Autodesk Fusion 360 part; units mm, degrees
note: some values were not read from the file. Chosen so that the rebuilt part matches the saved one: that a step has no effect.
(part 2 of 7)
  spline S227 degree 3 poles (-13.8567, 29.1803) (-14.5987, 29.1836) (-15.3407, 29.1895) (-16.0827, 29.1978) knots 0 0 0 0 1 1 1 1
  spline S228 degree 3 poles (-16.0827, 29.1978) (-16.65, 29.2012) (-16.65, 29.2012) (-17.2288, 29.2046) knots 0 0 0 0 1 1 1 1
  spline S229 degree 3 poles (-17.2288, 29.2046) (-18.1659, 29.2105) (-19.1029, 29.2194) (-20.04, 29.2289) knots 0 0 0 0 1 1 1 1
  spline S230 degree 3 poles (-20.04, 29.2289) (-20.2868, 29.9693) (-20.2868, 29.9693) (-20.5385, 30.7246) knots 0 0 0 0 1 1 1 1
  spline S231 degree 3 poles (-20.5385, 30.7246) (-20.374, 31.0537) (-20.2095, 31.3827) (-20.04, 31.7217) knots 0 0 0 0 1 1 1 1
  spline S232 degree 3 poles (-20.04, 31.7217) (-19.7109, 31.7217) (-19.3819, 31.7217) (-19.0429, 31.7217) knots 0 0 0 0 1 1 1 1
  spline S233 degree 3 poles (-19.0429, 31.7217) (-18.7888, 33.3829) (-18.5414, 35.045) (-18.295, 36.7073) knots 0 0 0 0 1 1 1 1
  spline S234 degree 3 poles (-18.295, 36.7073) (-18.2237, 37.1732) (-18.1524, 37.6392) (-18.0789, 38.1192) knots 0 0 0 0 1 1 1 1
  spline S235 degree 3 poles (-18.0789, 38.1192) (-17.6788, 40.8437) (-17.4748, 43.4272) (-17.5472, 46.1798) knots 0 0 0 0 1 1 1 1
  spline S236 degree 3 poles (-17.5472, 46.1798) (-17.5472, 46.8379) (-17.5472, 47.496) (-17.5472, 48.1741) knots 0 0 0 0 1 1 1 1
  spline S237 degree 3 poles (-17.5472, 48.1741) (-16.019, 48.9382) (-14.4225, 48.7239) (-12.7486, 48.7038) knots 0 0 0 0 1 1 1 1
  spline S238 degree 3 poles (18.3488, 14.7708) (18.5134, 14.2772) (18.6779, 13.7837) (18.8474, 13.2751) knots 0 0 0 0 1 1 1 1
  spline S239 degree 3 poles (18.8474, 13.2751) (19.1764, 13.5219) (19.5055, 13.7687) (19.8445, 14.023) knots 0 0 0 0 1 1 1 1
  spline S240 degree 3 poles (19.8445, 14.023) (21.7354, 14.9684) (23.2516, 15.2282) (25.3286, 14.7708) knots 0 0 0 0 1 1 1 1
  spline S241 degree 3 poles (25.3286, 14.7708) (26.9337, 13.5072) (27.674, 12.7203) (28.32, 10.7824) knots 0 0 0 0 1 1 1 1
  spline S242 degree 3 poles (28.32, 10.7824) (28.4814, 7.8759) (28.2625, 5.9661) (26.4192, 3.6779) knots 0 0 0 0 1 1 1 1
  spline S243 degree 3 poles (26.4192, 3.6779) (25.1645, 2.6742) (24.4352, 2.3869) (22.8358, 2.3069) knots 0 0 0 0 1 1 1 1
  spline S244 degree 3 poles (22.8358, 2.3069) (21.7141, 2.5562) (21.7141, 2.5562) (20.8416, 3.304) knots 0 0 0 0 1 1 1 1
  spline S245 degree 3 poles (20.8416, 3.304) (20.3431, 4.9867) (20.3431, 4.9867) (20.3431, 6.7939) knots 0 0 0 0 1 1 1 1
  spline S246 degree 3 poles (20.3431, 6.7939) (21.2467, 8.0091) (21.2467, 8.0091) (22.3373, 8.7881) knots 0 0 0 0 1 1 1 1
  spline S247 degree 3 poles (22.3373, 8.7881) (22.6663, 8.7881) (22.9954, 8.7881) (23.3344, 8.7881) knots 0 0 0 0 1 1 1 1
  spline S248 degree 3 poles (23.3344, 8.7881) (23.3344, 9.2817) (23.3344, 9.7753) (23.3344, 10.2838) knots 0 0 0 0 1 1 1 1
  spline S249 degree 3 poles (23.3344, 10.2838) (20.7001, 10.0772) (19.1909, 9.7296) (17.3517, 7.791) knots 0 0 0 0 1 1 1 1
  spline S250 degree 3 poles (17.3517, 7.791) (16.5889, 6.5011) (15.9688, 5.1693) (15.3575, 3.8026) knots 0 0 0 0 1 1 1 1
  spline S251 degree 3 poles (15.3575, 3.8026) (15.0279, 3.1365) (14.6963, 2.4713) (14.3604, 1.8084) knots 0 0 0 0 1 1 1 1
  spline S252 degree 3 poles (14.3604, 1.8084) (14.3332, 2.5144) (14.314, 3.2208) (14.2981, 3.9272) knots 0 0 0 0 1 1 1 1
  spline S253 degree 3 poles (14.2981, 3.9272) (14.2865, 4.3205) (14.2749, 4.7138) (14.263, 5.1191) knots 0 0 0 0 1 1 1 1
  spline S254 degree 3 poles (14.263, 5.1191) (14.416, 6.9678) (15.057, 7.9891) (16.3546, 9.2867) knots 0 0 0 0 1 1 1 1
  spline S255 degree 3 poles (16.3546, 9.2867) (15.6742, 10.3876) (15.6742, 10.3876) (14.3604, 11.2809) knots 0 0 0 0 1 1 1 1
  spline S256 degree 3 poles (14.3604, 11.2809) (12.6618, 11.462) (11.0907, 11.3712) (9.3748, 11.2809) knots 0 0 0 0 1 1 1 1
  spline S257 degree 3 poles (9.3748, 11.2809) (9.3748, 8.9776) (9.3748, 6.6743) (9.3748, 4.3011) knots 0 0 0 0 1 1 1 1
  spline S258 degree 3 poles (9.3748, 4.3011) (9.0458, 4.3011) (8.7167, 4.3011) (8.3777, 4.3011) knots 0 0 0 0 1 1 1 1
  spline S259 degree 3 poles (8.3777, 4.3011) (8.5422, 6.769) (8.7068, 9.2368) (8.8763, 11.7795) knots 0 0 0 0 1 1 1 1
  spline S260 degree 3 poles (8.8763, 11.7795) (9.5446, 11.9954) (10.213, 12.2114) (10.9016, 12.4338) knots 0 0 0 0 1 1 1 1
  spline S261 degree 3 poles (10.9016, 12.4338) (12.4032, 12.9304) (13.853, 13.4679) (15.2952, 14.1165) knots 0 0 0 0 1 1 1 1
  spline S262 degree 3 poles (15.2952, 14.1165) (16.8532, 14.7708) (16.8532, 14.7708) (18.3488, 14.7708) knots 0 0 0 0 1 1 1 1
  line L8 (-26.0227, -2.6786) -> (-27.0198, -2.1801)
  spline S263 degree 3 poles (-29.014, 5.7968) (-28.8495, 5.7968) (-28.6849, 5.7968) (-28.5154, 5.7968) knots 0 0 0 0 1 1 1 1
  spline S264 degree 3 poles (-28.5154, 5.7968) (-28.9168, 2.7868) (-29.4551, -0.1922) (-30.0111, -3.1772) knots 0 0 0 0 1 1 1 1
  spline S265 degree 3 poles (-30.0111, -3.1772) (-30.3401, -3.1772) (-30.6692, -3.1772) (-31.0082, -3.1772) knots 0 0 0 0 1 1 1 1
  spline S266 degree 3 poles (-31.0082, -3.1772) (-31.1727, -4.1643) (-31.3373, -5.1515) (-31.5068, -6.1685) knots 0 0 0 0 1 1 1 1
  spline S267 degree 3 poles (-31.5068, -6.1685) (-31.1777, -6.1685) (-30.8487, -6.1685) (-30.5097, -6.1685) knots 0 0 0 0 1 1 1 1
  spline S268 degree 3 poles (-30.5097, -6.1685) (-30.3965, -5.7778) (-30.2834, -5.3871) (-30.1669, -4.9845) knots 0 0 0 0 1 1 1 1
  spline S269 degree 3 poles (-30.1669, -4.9845) (-29.5125, -3.6758) (-29.5125, -3.6758) (-28.2038, -3.0214) knots 0 0 0 0 1 1 1 1
  spline S270 degree 3 poles (-28.2038, -3.0214) (-27.8131, -2.9083) (-27.4223, -2.7952) (-27.0198, -2.6786) knots 0 0 0 0 1 1 1 1
  spline S271 degree 3 poles (-27.0198, -2.6786) (-27.0198, -3.1722) (-27.0198, -3.6658) (-27.0198, -4.1743) knots 0 0 0 0 1 1 1 1
  spline S272 degree 3 poles (-27.0198, -4.1743) (-26.1971, -3.5162) (-25.3745, -2.8581) (-24.527, -2.1801) knots 0 0 0 0 1 1 1 1
  spline S273 degree 3 poles (-24.527, -2.1801) (-24.1979, -2.3446) (-23.8689, -2.5091) (-23.5299, -2.6786) knots 0 0 0 0 1 1 1 1
  spline S274 degree 3 poles (-23.5299, -2.6786) (-23.6321, -3.034) (-23.7342, -3.3894) (-23.8395, -3.7556) knots 0 0 0 0 1 1 1 1
  spline S275 degree 3 poles (-23.8395, -3.7556) (-24.5799, -6.3878) (-25.222, -8.9341) (-25.5241, -11.6527) knots 0 0 0 0 1 1 1 1
  spline S276 degree 3 poles (-25.5241, -11.6527) (-24.7837, -11.8994) (-24.7837, -11.8994) (-24.0284, -12.1512) knots 0 0 0 0 1 1 1 1
  spline S277 degree 3 poles (-24.0284, -12.1512) (-24.193, -12.6448) (-24.3575, -13.1383) (-24.527, -13.6469) knots 0 0 0 0 1 1 1 1
  spline S278 degree 3 poles (-24.527, -13.6469) (-27.8175, -13.6469) (-31.1079, -13.6469) (-34.4981, -13.6469) knots 0 0 0 0 1 1 1 1
  spline S279 degree 3 poles (-34.4981, -13.6469) (-35.0613, -11.3941) (-34.8788, -11.0226) (-33.9995, -8.9729) knots 0 0 0 0 1 1 1 1
  spline S280 degree 3 poles (-33.9995, -8.9729) (-32.7046, -5.7885) (-31.6338, -2.5614) (-30.6031, 0.7178) knots 0 0 0 0 1 1 1 1
  spline S281 degree 3 poles (-30.6031, 0.7178) (-30.4466, 1.2151) (-30.2902, 1.7125) (-30.1289, 2.2249) knots 0 0 0 0 1 1 1 1
  spline S282 degree 3 poles (-30.1289, 2.2249) (-29.7557, 3.415) (-29.384, 4.6056) (-29.014, 5.7968) knots 0 0 0 0 1 1 1 1
  spline S283 degree 3 poles (-6.579, 14.2723) (-6.8553, 10.6585) (-7.9211, 7.4645) (-9.1029, 4.0519) knots 0 0 0 0 1 1 1 1
  spline S284 degree 3 poles (-9.1029, 4.0519) (-9.2909, 3.4992) (-9.4789, 2.9465) (-9.6725, 2.377) knots 0 0 0 0 1 1 1 1
  spline S285 degree 3 poles (-9.6725, 2.377) (-10.1336, 1.023) (-10.5982, -0.3298) (-11.066, -1.6815) knots 0 0 0 0 1 1 1 1
  spline S286 degree 3 poles (-11.066, -1.6815) (-11.2305, -1.6815) (-11.395, -1.6815) (-11.5645, -1.6815) knots 0 0 0 0 1 1 1 1
  spline S287 degree 3 poles (-11.5645, -1.6815) (-12.3656, 1.5954) (-11.5813, 4.1249) (-10.5674, 7.2925) knots 0 0 0 0 1 1 1 1
  spline S288 degree 3 poles (-10.5674, 7.2925) (-11.8836, 7.6215) (-13.1998, 7.9506) (-14.5559, 8.2896) knots 0 0 0 0 1 1 1 1
  spline S289 degree 3 poles (-14.5559, 8.2896) (-14.633, 7.287) (-14.633, 7.287) (-14.7117, 6.2642) knots 0 0 0 0 1 1 1 1
  spline S290 degree 3 poles (-14.7117, 6.2642) (-14.9562, 4.0103) (-15.5889, 2.3551) (-16.5501, 0.3127) knots 0 0 0 0 1 1 1 1
  spline S291 degree 3 poles (-16.5501, 0.3127) (-16.6735, -0.1963) (-16.6735, -0.1963) (-16.7994, -0.7156) knots 0 0 0 0 1 1 1 1
  spline S292 degree 3 poles (-16.7994, -0.7156) (-17.1673, -2.1414) (-17.8648, -3.3729) (-18.5443, -4.6729) knots 0 0 0 0 1 1 1 1
  spline S293 degree 3 poles (-18.5443, -4.6729) (-18.8734, -4.6729) (-19.2024, -4.6729) (-19.5414, -4.6729) knots 0 0 0 0 1 1 1 1
  spline S294 degree 3 poles (-19.5414, -4.6729) (-19.7059, -5.0019) (-19.8705, -5.331) (-20.04, -5.67) knots 0 0 0 0 1 1 1 1
  spline S295 degree 3 poles (-20.04, -5.67) (-19.8124, -3.7358) (-19.3369, -1.9805) (-18.7118, -0.145) knots 0 0 0 0 1 1 1 1
  spline S296 degree 3 poles (-18.7118, -0.145) (-18.4747, 0.5525) (-18.4747, 0.5525) (-18.2327, 1.264) knots 0 0 0 0 1 1 1 1
  spline S297 degree 3 poles (-18.2327, 1.264) (-17.9017, 2.2253) (-17.5655, 3.1848) (-17.2239, 4.1424) knots 0 0 0 0 1 1 1 1
  spline S298 degree 3 poles (-17.2239, 4.1424) (-16.167, 7.2893) (-15.9381, 9.5047) (-16.5501, 12.7766) knots 0 0 0 0 1 1 1 1
  spline S299 degree 3 poles (-16.5501, 12.7766) (-9.7531, 14.4937) (-9.7531, 14.4937) (-6.579, 14.2723) knots 0 0 0 0 1 1 1 1
  spline S300 degree 3 poles (20.8416, 47.6755) (28.3298, 48.1042) (28.3298, 48.1042) (30.1895, 46.6784) knots 0 0 0 0 1 1 1 1
  spline S301 degree 3 poles (30.1895, 46.6784) (32.0534, 44.1933) (33.0292, 42.0921) (32.6512, 38.9508) knots 0 0 0 0 1 1 1 1
  spline S302 degree 3 poles (32.6512, 38.9508) (32.538, 38.3749) (32.4249, 37.7991) (32.3084, 37.2058) knots 0 0 0 0 1 1 1 1
  spline S303 degree 3 poles (32.3084, 37.2058) (31.9794, 37.2058) (31.6503, 37.2058) (31.3113, 37.2058) knots 0 0 0 0 1 1 1 1
  spline S304 degree 3 poles (31.3113, 37.2058) (30.9822, 36.2187) (30.6532, 35.2316) (30.3142, 34.2145) knots 0 0 0 0 1 1 1 1
  spline S305 degree 3 poles (30.3142, 34.2145) (29.4916, 34.05) (28.6689, 33.8855) (27.8214, 33.7159) knots 0 0 0 0 1 1 1 1
  spline S306 degree 3 poles (27.8214, 33.7159) (27.8214, 33.3869) (27.8214, 33.0578) (27.8214, 32.7188) knots 0 0 0 0 1 1 1 1
  spline S307 degree 3 poles (27.8214, 32.7188) (27.4923, 32.8834) (27.1633, 33.0479) (26.8243, 33.2174) knots 0 0 0 0 1 1 1 1
  spline S308 degree 3 poles (26.8243, 33.2174) (26.9888, 33.711) (27.1533, 34.2045) (27.3228, 34.7131) knots 0 0 0 0 1 1 1 1
  spline S309 degree 3 poles (27.3228, 34.7131) (26.3357, 34.2195) (26.3357, 34.2195) (25.3286, 33.7159) knots 0 0 0 0 1 1 1 1
  spline S310 degree 3 poles (25.3286, 33.7159) (25.3826, 34.2143) (25.3826, 34.2143) (25.4377, 34.7228) knots 0 0 0 0 1 1 1 1
  spline S311 degree 3 poles (25.4377, 34.7228) (25.7733, 38.0559) (25.8855, 41.3354) (25.8272, 44.6842) knots 0 0 0 0 1 1 1 1
  spline S312 degree 3 poles (25.8272, 44.6842) (25.3336, 44.8487) (24.84, 45.0132) (24.3315, 45.1827) knots 0 0 0 0 1 1 1 1
  spline S313 degree 3 poles (24.3315, 45.1827) (24.167, 45.5118) (24.0025, 45.8408) (23.8329, 46.1798) knots 0 0 0 0 1 1 1 1
  spline S314 degree 3 poles (23.8329, 46.1798) (22.8464, 46.5423) (21.8489, 46.8769) (20.8416, 47.177) knots 0 0 0 0 1 1 1 1
  spline S315 degree 3 poles (20.8416, 47.177) (20.8416, 47.3415) (20.8416, 47.506) (20.8416, 47.6755) knots 0 0 0 0 1 1 1 1
  spline S316 degree 3 poles (38.2911, 14.2723) (38.0022, 11.1132) (37.2607, 8.3042) (36.2657, 5.2983) knots 0 0 0 0 1 1 1 1
  spline S317 degree 3 poles (36.2657, 5.2983) (36.1253, 4.8644) (35.9848, 4.4306) (35.8402, 3.9837) knots 0 0 0 0 1 1 1 1
  spline S318 degree 3 poles (35.8402, 3.9837) (35.497, 2.9251) (35.1506, 1.8677) (34.8012, 0.8112) knots 0 0 0 0 1 1 1 1
  spline S319 degree 3 poles (34.8012, 0.8112) (34.6367, 0.8112) (34.4721, 0.8112) (34.3026, 0.8112) knots 0 0 0 0 1 1 1 1
  spline S320 degree 3 poles (34.3026, 0.8112) (34.1381, 2.292) (33.9736, 3.7727) (33.8041, 5.2983) knots 0 0 0 0 1 1 1 1
  spline S321 degree 3 poles (33.8041, 5.2983) (33.3105, 5.4628) (32.8169, 5.6273) (32.3084, 5.7968) knots 0 0 0 0 1 1 1 1
  spline S322 degree 3 poles (32.3084, 5.7968) (32.1439, 5.4678) (31.9794, 5.1387) (31.8098, 4.7997) knots 0 0 0 0 1 1 1 1
  spline S323 degree 3 poles (31.8098, 4.7997) (31.4808, 4.7997) (31.1517, 4.7997) (30.8127, 4.7997) knots 0 0 0 0 1 1 1 1
  spline S324 degree 3 poles (30.8127, 4.7997) (30.6482, 5.2933) (30.4837, 5.7868) (30.3142, 6.2954) knots 0 0 0 0 1 1 1 1
  spline S325 degree 3 poles (30.3142, 6.2954) (30.1497, 5.8018) (29.9851, 5.3082) (29.8156, 4.7997) knots 0 0 0 0 1 1 1 1
  spline S326 degree 3 poles (29.8156, 4.7997) (28.7873, 3.9584) (28.7873, 3.9584) (27.8214, 3.304) knots 0 0 0 0 1 1 1 1
  spline S327 degree 3 poles (27.8214, 3.304) (27.8992, 3.5759) (27.9769, 3.8477) (28.057, 4.1278) knots 0 0 0 0 1 1 1 1
  spline S328 degree 3 poles (28.057, 4.1278) (28.81, 7.045) (28.7919, 9.3045) (28.32, 12.278) knots 0 0 0 0 1 1 1 1
  spline S329 degree 3 poles (28.32, 12.278) (31.4839, 13.7069) (34.818, 14.4504) (38.2911, 14.2723) knots 0 0 0 0 1 1 1 1
  spline S330 degree 3 poles (26.3257, 45.1827) (26.3829, 41.4883) (26.2817, 37.8828) (25.8272, 34.2145) knots 0 0 0 0 1 1 1 1
  spline S331 degree 3 poles (25.8272, 34.2145) (26.3207, 34.379) (26.8143, 34.5435) (27.3228, 34.7131) knots 0 0 0 0 1 1 1 1
  spline S332 degree 3 poles (27.3228, 34.7131) (27.4874, 34.055) (27.6519, 33.3969) (27.8214, 32.7188) knots 0 0 0 0 1 1 1 1
  spline S333 degree 3 poles (27.8214, 32.7188) (27.8214, 33.0479) (27.8214, 33.3769) (27.8214, 33.7159) knots 0 0 0 0 1 1 1 1
  spline S334 degree 3 poles (27.8214, 33.7159) (28.2019, 33.9422) (28.5823, 34.1684) (28.9743, 34.4015) knots 0 0 0 0 1 1 1 1
  spline S335 degree 3 poles (28.9743, 34.4015) (30.3185, 35.2142) (30.9597, 35.9083) (31.8098, 37.2058) knots 0 0 0 0 1 1 1 1
  spline S336 degree 3 poles (31.8098, 37.2058) (31.6498, 34.5644) (30.2104, 32.9347) (28.32, 31.2232) knots 0 0 0 0 1 1 1 1
  spline S337 degree 3 poles (28.32, 31.2232) (25.2863, 29.2842) (22.4551, 28.4938) (18.8474, 28.7304) knots 0 0 0 0 1 1 1 1
  spline S338 degree 3 poles (18.8474, 28.7304) (16.6791, 29.2211) (14.8803, 29.6746) (13.3321, 31.3166) knots 0 0 0 0 1 1 1 1
  spline S339 degree 3 poles (13.3321, 31.3166) (13.1779, 31.6148) (13.0236, 31.913) (12.8647, 32.2203) knots 0 0 0 0 1 1 1 1
  spline S340 degree 3 poles (12.8647, 32.2203) (13.3583, 32.2203) (13.8519, 32.2203) (14.3604, 32.2203) knots 0 0 0 0 1 1 1 1
  spline S341 degree 3 poles (14.3604, 32.2203) (14.5249, 31.8912) (14.6894, 31.5622) (14.8589, 31.2232) knots 0 0 0 0 1 1 1 1
  spline S342 degree 3 poles (14.8589, 31.2232) (15.188, 31.2232) (15.517, 31.2232) (15.8561, 31.2232) knots 0 0 0 0 1 1 1 1
  spline S343 degree 3 poles (15.8561, 31.2232) (15.9404, 32.2513) (16.0232, 33.2796) (16.1053, 34.308) knots 0 0 0 0 1 1 1 1
  spline S344 degree 3 poles (16.1053, 34.308) (16.1516, 34.8806) (16.1979, 35.4532) (16.2455, 36.0432) knots 0 0 0 0 1 1 1 1
  spline S345 degree 3 poles (16.2455, 36.0432) (16.3918, 37.6505) (16.3918, 37.6505) (16.2455, 39.0384) knots 0 0 0 0 1 1 1 1
  spline S346 degree 3 poles (16.2455, 39.0384) (16.3966, 40.6435) (17.1498, 41.1797) (18.3488, 42.1914) knots 0 0 0 0 1 1 1 1
  spline S347 degree 3 poles (18.3488, 42.1914) (18.2775, 41.6043) (18.2775, 41.6043) (18.2047, 41.0054) knots 0 0 0 0 1 1 1 1
  spline S348 degree 3 poles (18.2047, 41.0054) (17.8829, 37.9552) (17.7361, 35.5952) (18.8474, 32.7188) knots 0 0 0 0 1 1 1 1
  spline S349 degree 3 poles (18.8474, 32.7188) (19.9685, 32.2858) (19.9685, 32.2858) (21.3402, 32.2203) knots 0 0 0 0 1 1 1 1
  spline S350 degree 3 poles (21.3402, 32.2203) (23.3479, 33.4343) (24.1093, 34.5169) (24.8301, 36.7073) knots 0 0 0 0 1 1 1 1
  spline S351 degree 3 poles (24.8301, 36.7073) (25.0733, 38.1949) (25.0733, 38.1949) (25.1728, 39.7298) knots 0 0 0 0 1 1 1 1
  spline S352 degree 3 poles (25.1728, 39.7298) (25.2159, 40.2394) (25.2589, 40.749) (25.3033, 41.2741) knots 0 0 0 0 1 1 1 1
  spline S353 degree 3 poles (25.3033, 41.2741) (25.326, 42.5423) (25.2125, 43.4849) (24.8301, 44.6842) knots 0 0 0 0 1 1 1 1
  spline S354 degree 3 poles (24.8301, 44.6842) (25.8272, 45.1827) (25.8272, 45.1827) (26.3257, 45.1827) knots 0 0 0 0 1 1 1 1
  spline S355 degree 3 poles (-55.936, 17.7622) (-54.9389, 16.9208) (-54.9389, 16.9208) (-54.4403, 15.7679) knots 0 0 0 0 1 1 1 1
  spline S356 degree 3 poles (-54.4403, 15.7679) (-54.4808, 14.1503) (-54.8175, 13.4312) (-55.8114, 12.1534) knots 0 0 0 0 1 1 1 1
  spline S357 degree 3 poles (-55.8114, 12.1534) (-57.0473, 11.1921) (-57.8858, 10.9535) (-59.4259, 10.7824) knots 0 0 0 0 1 1 1 1
  spline S358 degree 3 poles (-59.4259, 10.7824) (-59.2614, 10.4533) (-59.0969, 10.1243) (-58.9274, 9.7853) knots 0 0 0 0 1 1 1 1
  spline S359 degree 3 poles (-58.9274, 9.7853) (-57.6112, 9.7853) (-56.295, 9.7853) (-54.9389, 9.7853) knots 0 0 0 0 1 1 1 1
  spline S360 degree 3 poles (-54.9389, 9.7853) (-54.9389, 9.4562) (-54.9389, 9.1272) (-54.9389, 8.7881) knots 0 0 0 0 1 1 1 1
  spline S361 degree 3 poles (-54.9389, 8.7881) (-56.4196, 8.6236) (-57.9003, 8.4591) (-59.4259, 8.2896) knots 0 0 0 0 1 1 1 1
  spline S362 degree 3 poles (-59.4259, 8.2896) (-59.5904, 7.467) (-59.755, 6.6444) (-59.9245, 5.7968) knots 0 0 0 0 1 1 1 1
  spline S363 degree 3 poles (-59.9245, 5.7968) (-58.9373, 5.9613) (-57.9502, 6.1259) (-56.9331, 6.2954) knots 0 0 0 0 1 1 1 1
  spline S364 degree 3 poles (-56.9331, 6.2954) (-56.7686, 5.9663) (-56.6041, 5.6373) (-56.4346, 5.2983) knots 0 0 0 0 1 1 1 1
  spline S365 degree 3 poles (-56.4346, 5.2983) (-54.9243, 4.9703) (-54.9243, 4.9703) (-53.4432, 4.7997) knots 0 0 0 0 1 1 1 1
  spline S366 degree 3 poles (-53.4432, 4.7997) (-53.4432, 4.6352) (-53.4432, 4.4706) (-53.4432, 4.3011) knots 0 0 0 0 1 1 1 1
  spline S367 degree 3 poles (-53.4432, 4.3011) (-56.3715, 4.1443) (-58.8427, 4.28) (-61.4201, 5.7968) knots 0 0 0 0 1 1 1 1
  spline S368 degree 3 poles (-61.4201, 5.7968) (-62.855, 7.3751) (-63.3516, 8.3646) (-63.6636, 10.4708) knots 0 0 0 0 1 1 1 1
  spline S369 degree 3 poles (-63.6636, 10.4708) (-63.2943, 13.1486) (-62.3353, 15.2566) (-60.5165, 17.2636) knots 0 0 0 0 1 1 1 1
  spline S370 degree 3 poles (-60.5165, 17.2636) (-58.8998, 18.0027) (-57.6862, 17.9849) (-55.936, 17.7622) knots 0 0 0 0 1 1 1 1
  spline S371 degree 3 poles (-45.9649, -0.6844) (-45.6358, -0.8489) (-45.3068, -1.0135) (-44.9678, -1.183) knots 0 0 0 0 1 1 1 1
  spline S372 degree 3 poles (-44.9678, -1.183) (-45.2845, -5.0064) (-47.6479, -6.7829) (-50.4519, -9.1599) knots 0 0 0 0 1 1 1 1
  spline S373 degree 3 poles (-50.4519, -9.1599) (-54.7143, -12.1512) (-54.7143, -12.1512) (-56.4346, -12.1512) knots 0 0 0 0 1 1 1 1
  spline S374 degree 3 poles (-56.4346, -12.1512) (-56.0918, -10.9671) (-56.0918, -10.9671) (-55.4375, -9.6584) knots 0 0 0 0 1 1 1 1
  spline S375 degree 3 poles (-55.4375, -9.6584) (-54.1911, -9.0664) (-54.1911, -9.0664) (-52.9447, -8.6613) knots 0 0 0 0 1 1 1 1
  spline S376 degree 3 poles (-52.9447, -8.6613) (-52.6156, -8.3323) (-52.2866, -8.0032) (-51.9476, -7.6642) knots 0 0 0 0 1 1 1 1
  spline S377 degree 3 poles (-51.9476, -7.6642) (-51.9476, -7.1706) (-51.9476, -6.6771) (-51.9476, -6.1685) knots 0 0 0 0 1 1 1 1
  spline S378 degree 3 poles (-51.9476, -6.1685) (-52.4411, -6.3331) (-52.9347, -6.4976) (-53.4432, -6.6671) knots 0 0 0 0 1 1 1 1
  spline S379 degree 3 poles (-53.4432, -6.6671) (-54.5338, -6.449) (-54.5338, -6.449) (-55.4375, -6.1685) knots 0 0 0 0 1 1 1 1
  spline S380 degree 3 poles (-55.4375, -6.1685) (-55.602, -6.6621) (-55.7665, -7.1557) (-55.936, -7.6642) knots 0 0 0 0 1 1 1 1
  spline S381 degree 3 poles (-55.936, -7.6642) (-56.9232, -7.6642) (-57.9103, -7.6642) (-58.9274, -7.6642) knots 0 0 0 0 1 1 1 1
  spline S382 degree 3 poles (-58.9274, -7.6642) (-59.0919, -7.9933) (-59.2564, -8.3223) (-59.4259, -8.6613) knots 0 0 0 0 1 1 1 1
  spline S383 degree 3 poles (-59.4259, -8.6613) (-59.4259, -8.3323) (-59.4259, -8.0032) (-59.4259, -7.6642) knots 0 0 0 0 1 1 1 1
  spline S384 degree 3 poles (-59.4259, -7.6642) (-59.8989, -7.6745) (-60.3719, -7.6848) (-60.8593, -7.6954) knots 0 0 0 0 1 1 1 1
  spline S385 degree 3 poles (-60.8593, -7.6954) (-62.4172, -7.6642) (-62.4172, -7.6642) (-63.4144, -7.1656) knots 0 0 0 0 1 1 1 1
  spline S386 degree 3 poles (-63.4144, -7.1656) (-63.4144, -6.8366) (-63.4144, -6.5076) (-63.4144, -6.1685) knots 0 0 0 0 1 1 1 1
  spline S387 degree 3 poles (-63.4144, -6.1685) (-63.7434, -6.1685) (-64.0724, -6.1685) (-64.4115, -6.1685) knots 0 0 0 0 1 1 1 1
  spline S388 degree 3 poles (-64.4115, -6.1685) (-64.2469, -5.8395) (-64.0824, -5.5104) (-63.9129, -5.1714) knots 0 0 0 0 1 1 1 1
  spline S389 degree 3 poles (-63.9129, -5.1714) (-63.4193, -5.3359) (-62.9258, -5.5005) (-62.4172, -5.67) knots 0 0 0 0 1 1 1 1
  spline S390 degree 3 poles (-62.4172, -5.67) (-56.3865, -6.2377) (-51.9342, -4.5069) (-46.9601, -1.22) knots 0 0 0 0 1 1 1 1
  spline S391 degree 3 poles (-46.9601, -1.22) (-46.6317, -1.0432) (-46.3032, -0.8665) (-45.9649, -0.6844) knots 0 0 0 0 1 1 1 1
  spline S392 degree 3 poles (-22.4081, 47.6755) (-21.7791, 47.3543) (-21.1533, 47.0261) (-20.5385, 46.6784) knots 0 0 0 0 1 1 1 1
  spline S393 degree 3 poles (-20.5385, 46.6784) (-20.5116, 45.8684) (-20.4923, 45.0582) (-20.4762, 44.2479) knots 0 0 0 0 1 1 1 1
  spline S394 degree 3 poles (-20.4762, 44.2479) (-20.4647, 43.7968) (-20.4531, 43.3456) (-20.4412, 42.8808) knots 0 0 0 0 1 1 1 1
  spline S395 degree 3 poles (-20.4412, 42.8808) (-20.5385, 41.6928) (-20.5385, 41.6928) (-21.5356, 40.6957) knots 0 0 0 0 1 1 1 1
  spline S396 degree 3 poles (-21.5356, 40.6957) (-22.5016, 40.6646) (-22.5016, 40.6646) (-23.5299, 41.1943) knots 0 0 0 0 1 1 1 1
  spline S397 degree 3 poles (-23.5299, 41.1943) (-24.0628, 42.3422) (-24.5628, 43.5062) (-25.0255, 44.6842) knots 0 0 0 0 1 1 1 1
  spline S398 degree 3 poles (-25.0255, 44.6842) (-26.2248, 45.2838) (-26.9948, 45.2329) (-28.3285, 45.2139) knots 0 0 0 0 1 1 1 1
  spline S399 degree 3 poles (-28.3285, 45.2139) (-28.7359, 45.2094) (-29.1434, 45.2049) (-29.5632, 45.2003) knots 0 0 0 0 1 1 1 1
  spline S400 degree 3 poles (-29.5632, 45.2003) (-29.8755, 45.1945) (-30.1879, 45.1887) (-30.5097, 45.1827) knots 0 0 0 0 1 1 1 1
  spline S401 degree 3 poles (-30.5097, 45.1827) (-31.2575, 43.7122) (-31.9057, 42.2338) (-32.5039, 40.6957) knots 0 0 0 0 1 1 1 1
  spline S402 degree 3 poles (-32.5039, 40.6957) (-33.096, 42.4055) (-32.9039, 43.3769) (-32.2858, 45.0581) knots 0 0 0 0 1 1 1 1
  spline S403 degree 3 poles (-32.2858, 45.0581) (-32.1424, 45.4565) (-31.9991, 45.855) (-31.8515, 46.2655) knots 0 0 0 0 1 1 1 1
  spline S404 degree 3 poles (-31.8515, 46.2655) (-31.6808, 46.7167) (-31.6808, 46.7167) (-31.5068, 47.177) knots 0 0 0 0 1 1 1 1
  spline S405 degree 3 poles (-31.5068, 47.177) (-32.4939, 47.0124) (-33.4811, 46.8479) (-34.4981, 46.6784) knots 0 0 0 0 1 1 1 1
  spline S406 degree 3 poles (-34.4981, 46.6784) (-31.002, 49.4512) (-26.4314, 49.4828) (-22.4081, 47.6755) knots 0 0 0 0 1 1 1 1
  spline S407 degree 3 poles (6.3835, 14.7708) (6.1117, 11.2375) (5.0827, 8.1261) (3.8907, 4.7997) knots 0 0 0 0 1 1 1 1
  spline S408 degree 3 poles (3.8907, 4.7997) (3.7262, 4.7997) (3.5617, 4.7997) (3.3922, 4.7997) knots 0 0 0 0 1 1 1 1
  spline S409 degree 3 poles (3.3922, 4.7997) (3.8725, 10.0635) (3.8725, 10.0635) (4.3893, 12.278) knots 0 0 0 0 1 1 1 1
  spline S410 degree 3 poles (4.3893, 12.278) (3.0731, 11.7845) (1.7569, 11.2909) (0.4008, 10.7824) knots 0 0 0 0 1 1 1 1
  spline S411 degree 3 poles (0.4008, 10.7824) (0.4008, 10.1243) (0.4008, 9.4662) (0.4008, 8.7881) knots 0 0 0 0 1 1 1 1
  spline S412 degree 3 poles (0.4008, 8.7881) (-0.2847, 7.9157) (-0.2847, 7.9157) (-1.0949, 7.2925) knots 0 0 0 0 1 1 1 1
  spline S413 degree 3 poles (-1.0949, 7.2925) (-1.4239, 7.2925) (-1.7529, 7.2925) (-2.092, 7.2925) knots 0 0 0 0 1 1 1 1
  spline S414 degree 3 poles (-2.092, 7.2925) (-2.092, 6.7989) (-2.092, 6.3053) (-2.092, 5.7968) knots 0 0 0 0 1 1 1 1
  spline S415 degree 3 poles (-2.092, 5.7968) (-1.5984, 5.6323) (-1.1048, 5.4678) (-0.5963, 5.2983) knots 0 0 0 0 1 1 1 1
  spline S416 degree 3 poles (-0.5963, 5.2983) (-0.9253, 5.1337) (-1.2544, 4.9692) (-1.5934, 4.7997) knots 0 0 0 0 1 1 1 1
  spline S417 degree 3 poles (-1.5934, 4.7997) (-1.9225, 4.9642) (-2.2515, 5.1287) (-2.5905, 5.2983) knots 0 0 0 0 1 1 1 1
  spline S418 degree 3 poles (-2.5905, 5.2983) (-2.6317, 4.9075) (-2.6728, 4.5168) (-2.7152, 4.1142) knots 0 0 0 0 1 1 1 1
  spline S419 degree 3 poles (-2.7152, 4.1142) (-3.0891, 2.8055) (-3.0891, 2.8055) (-4.1096, 2.2251) knots 0 0 0 0 1 1 1 1
  spline S420 degree 3 poles (-4.1096, 2.2251) (-4.5916, 2.0188) (-4.5916, 2.0188) (-5.0833, 1.8084) knots 0 0 0 0 1 1 1 1
  spline S421 degree 3 poles (-5.0833, 1.8084) (-4.9213, 2.3067) (-4.9213, 2.3067) (-4.7561, 2.8152) knots 0 0 0 0 1 1 1 1
  spline S422 degree 3 poles (-4.7561, 2.8152) (-3.7278, 6.219) (-3.4024, 9.2301) (-3.5876, 12.7766) knots 0 0 0 0 1 1 1 1
  spline S423 degree 3 poles (-3.5876, 12.7766) (-3.1011, 12.8788) (-2.6146, 12.981) (-2.1134, 13.0862) knots 0 0 0 0 1 1 1 1
  spline S424 degree 3 poles (-2.1134, 13.0862) (-1.4791, 13.2206) (-0.8448, 13.3549) (-0.1912, 13.4933) knots 0 0 0 0 1 1 1 1
  spline S425 degree 3 poles (-0.1912, 13.4933) (0.4392, 13.6263) (1.0697, 13.7593) (1.7193, 13.8964) knots 0 0 0 0 1 1 1 1
  spline S426 degree 3 poles (1.7193, 13.8964) (5.6111, 14.7708) (5.6111, 14.7708) (6.3835, 14.7708) knots 0 0 0 0 1 1 1 1
  spline S427 degree 3 poles (4.3893, 12.278) (3.9089, 7.0142) (3.9089, 7.0142) (3.3922, 4.7997) knots 0 0 0 0 1 1 1 1
  spline S428 degree 3 poles (3.3922, 4.7997) (3.0631, 4.7997) (2.7341, 4.7997) (2.395, 4.7997) knots 0 0 0 0 1 1 1 1
  spline S429 degree 3 poles (2.395, 4.7997) (2.2305, 4.4706) (2.066, 4.1416) (1.8965, 3.8026) knots 0 0 0 0 1 1 1 1
  spline S430 degree 3 poles (1.8965, 3.8026) (1.0719, 3.6073) (0.2396, 3.4433) (-0.5963, 3.304) knots 0 0 0 0 1 1 1 1
  spline S431 degree 3 poles (-0.5963, 3.304) (-1.0899, 3.1395) (-1.5834, 2.975) (-2.092, 2.8055) knots 0 0 0 0 1 1 1 1
  spline S432 degree 3 poles (-2.092, 2.8055) (-2.092, 3.4636) (-2.092, 4.1217) (-2.092, 4.7997) knots 0 0 0 0 1 1 1 1
  spline S433 degree 3 poles (-2.092, 4.7997) (-1.7629, 4.9642) (-1.4339, 5.1287) (-1.0949, 5.2983) knots 0 0 0 0 1 1 1 1
  spline S434 degree 3 poles (-1.0949, 5.2983) (-1.4239, 5.4628) (-1.7529, 5.6273) (-2.092, 5.7968) knots 0 0 0 0 1 1 1 1
  spline S435 degree 3 poles (-2.092, 5.7968) (-2.092, 6.2904) (-2.092, 6.7839) (-2.092, 7.2925) knots 0 0 0 0 1 1 1 1
  spline S436 degree 3 poles (-2.092, 7.2925) (-1.7629, 7.2925) (-1.4339, 7.2925) (-1.0949, 7.2925) knots 0 0 0 0 1 1 1 1
  spline S437 degree 3 poles (-1.0949, 7.2925) (-0.9303, 7.786) (-0.7658, 8.2796) (-0.5963, 8.7881) knots 0 0 0 0 1 1 1 1
  spline S438 degree 3 poles (-0.5963, 8.7881) (-0.2673, 8.7881) (0.0618, 8.7881) (0.4008, 8.7881) knots 0 0 0 0 1 1 1 1
  spline S439 degree 3 poles (0.4008, 8.7881) (0.4008, 9.4462) (0.4008, 10.1043) (0.4008, 10.7824) knots 0 0 0 0 1 1 1 1
  spline S440 degree 3 poles (0.4008, 10.7824) (0.0718, 10.9469) (-0.2573, 11.1114) (-0.5963, 11.2809) knots 0 0 0 0 1 1 1 1
  spline S441 degree 3 poles (-0.5963, 11.2809) (1.2083, 11.9372) (2.4427, 12.278) (4.3893, 12.278) knots 0 0 0 0 1 1 1 1
  spline S442 degree 3 poles (14.8589, 41.6928) (16.0929, 41.1993) (16.0929, 41.1993) (17.3517, 40.6957) knots 0 0 0 0 1 1 1 1
  spline S443 degree 3 poles (17.3517, 40.6957) (17.2752, 40.2729) (17.1988, 39.85) (17.12, 39.4143) knots 0 0 0 0 1 1 1 1
  spline S444 degree 3 poles (17.12, 39.4143) (16.8524, 37.6994) (16.6964, 36.0077) (16.5727, 34.2768) knots 0 0 0 0 1 1 1 1
  spline S445 degree 3 poles (16.5727, 34.2768) (16.531, 33.7023) (16.4892, 33.1277) (16.4461, 32.5358) knots 0 0 0 0 1 1 1 1
  spline S446 degree 3 poles (16.4461, 32.5358) (16.4159, 32.1026) (16.3857, 31.6694) (16.3546, 31.2232) knots 0 0 0 0 1 1 1 1
  spline S447 degree 3 poles (16.3546, 31.2232) (15.6965, 31.2232) (15.0384, 31.2232) (14.3604, 31.2232) knots 0 0 0 0 1 1 1 1
  spline S448 degree 3 poles (14.3604, 31.2232) (14.3604, 31.5522) (14.3604, 31.8813) (14.3604, 32.2203) knots 0 0 0 0 1 1 1 1
  spline S449 degree 3 poles (14.3604, 32.2203) (13.5378, 32.2203) (12.7151, 32.2203) (11.8676, 32.2203) knots 0 0 0 0 1 1 1 1
  spline S450 degree 3 poles (11.8676, 32.2203) (12.0321, 33.2074) (12.1966, 34.1946) (12.3662, 35.2116) knots 0 0 0 0 1 1 1 1
  spline S451 degree 3 poles (12.3662, 35.2116) (12.0371, 35.2116) (11.7081, 35.2116) (11.369, 35.2116) knots 0 0 0 0 1 1 1 1
  spline S452 degree 3 poles (11.369, 35.2116) (11.369, 36.6923) (11.369, 38.173) (11.369, 39.6986) knots 0 0 0 0 1 1 1 1
  spline S453 degree 3 poles (11.369, 39.6986) (11.6981, 39.0405) (12.0271, 38.3824) (12.3662, 37.7044) knots 0 0 0 0 1 1 1 1
  spline S454 degree 3 poles (12.3662, 37.7044) (12.8597, 37.8689) (13.3533, 38.0334) (13.8618, 38.2029) knots 0 0 0 0 1 1 1 1
  spline S455 degree 3 poles (13.8618, 38.2029) (13.8618, 38.532) (13.8618, 38.861) (13.8618, 39.2001) knots 0 0 0 0 1 1 1 1
  spline S456 degree 3 poles (13.8618, 39.2001) (14.1909, 39.2001) (14.5199, 39.2001) (14.8589, 39.2001) knots 0 0 0 0 1 1 1 1
  spline S457 degree 3 poles (14.8589, 39.2001) (14.8589, 40.0227) (14.8589, 40.8453) (14.8589, 41.6928) knots 0 0 0 0 1 1 1 1
  spline S458 degree 3 poles (24.3315, 13.7737) (25.3286, 13.7737) (25.3286, 13.7737) (26.388, 13.1193) knots 0 0 0 0 1 1 1 1
  spline S459 degree 3 poles (26.388, 13.1193) (27.8513, 11.0221) (27.5634, 8.7802) (27.3228, 6.2954) knots 0 0 0 0 1 1 1 1
  spline S460 degree 3 poles (27.3228, 6.2954) (27.1583, 5.9663) (26.9938, 5.6373) (26.8243, 5.2983) knots 0 0 0 0 1 1 1 1
  spline S461 degree 3 poles (26.8243, 5.2983) (26.4952, 5.2263) (26.1662, 5.1543) (25.8272, 5.0801) knots 0 0 0 0 1 1 1 1
  spline S462 degree 3 poles (25.8272, 5.0801) (25.4981, 4.9876) (25.1691, 4.895) (24.8301, 4.7997) knots 0 0 0 0 1 1 1 1
  spline S463 degree 3 poles (24.8301, 4.7997) (24.6655, 4.3061) (24.501, 3.8126) (24.3315, 3.304) knots 0 0 0 0 1 1 1 1
  spline S464 degree 3 poles (24.3315, 3.304) (23.3444, 3.304) (22.3572, 3.304) (21.3402, 3.304) knots 0 0 0 0 1 1 1 1
  spline S465 degree 3 poles (21.3402, 3.304) (21.1532, 4.6439) (21.1532, 4.6439) (21.3402, 6.2954) knots 0 0 0 0 1 1 1 1
  spline S466 degree 3 poles (21.3402, 6.2954) (21.844, 6.6758) (22.3479, 7.0563) (22.867, 7.4483) knots 0 0 0 0 1 1 1 1
  spline S467 degree 3 poles (22.867, 7.4483) (24.451, 8.5859) (24.451, 8.5859) (24.4016, 9.9235) knots 0 0 0 0 1 1 1 1
  spline S468 degree 3 poles (24.4016, 9.9235) (24.2945, 10.7306) (24.1609, 11.5348) (23.9985, 12.3326) knots 0 0 0 0 1 1 1 1
  spline S469 degree 3 poles (23.9985, 12.3326) (23.9165, 12.7991) (23.9165, 12.7991) (23.8329, 13.2751) knots 0 0 0 0 1 1 1 1
  spline S470 degree 3 poles (23.8329, 13.2751) (23.9975, 13.4397) (24.162, 13.6042) (24.3315, 13.7737) knots 0 0 0 0 1 1 1 1
  spline S471 degree 3 poles (7.8792, 42.1914) (8.0437, 42.1914) (8.2082, 42.1914) (8.3777, 42.1914) knots 0 0 0 0 1 1 1 1
  spline S472 degree 3 poles (8.3777, 42.1914) (7.9267, 35.8102) (7.9267, 35.8102) (7.5676, 33.7159) knots 0 0 0 0 1 1 1 1
  spline S473 degree 3 poles (7.5676, 33.7159) (7.3813, 32.226) (7.5387, 31.1746) (7.8792, 29.7275) knots 0 0 0 0 1 1 1 1
  spline S474 degree 3 poles (7.8792, 29.7275) (7.3806, 29.2289) (7.3806, 29.2289) (5.587, 29.1803) knots 0 0 0 0 1 1 1 1
  spline S475 degree 3 poles (5.587, 29.1803) (4.845, 29.1836) (4.103, 29.1895) (3.361, 29.1978) knots 0 0 0 0 1 1 1 1
  spline S476 degree 3 poles (3.361, 29.1978) (2.9828, 29.2) (2.6046, 29.2023) (2.2149, 29.2046) knots 0 0 0 0 1 1 1 1
  spline S477 degree 3 poles (2.2149, 29.2046) (1.2778, 29.2105) (0.3408, 29.2194) (-0.5963, 29.2289) knots 0 0 0 0 1 1 1 1
  spline S478 degree 3 poles (-0.5963, 29.2289) (-0.5963, 30.999) (-0.4762, 31.7728) (0.1515, 33.342) knots 0 0 0 0 1 1 1 1
  spline S479 degree 3 poles (0.1515, 33.342) (0.2904, 33.6942) (0.4292, 34.0464) (0.5722, 34.4092) knots 0 0 0 0 1 1 1 1
  spline S480 degree 3 poles (0.5722, 34.4092) (0.7341, 34.8064) (0.7341, 34.8064) (0.8994, 35.2116) knots 0 0 0 0 1 1 1 1
  spline S481 degree 3 poles (0.8994, 35.2116) (1.0639, 35.2116) (1.2284, 35.2116) (1.3979, 35.2116) knots 0 0 0 0 1 1 1 1
  spline S482 degree 3 poles (1.3979, 35.2116) (1.5624, 33.8954) (1.727, 32.5792) (1.8965, 31.2232) knots 0 0 0 0 1 1 1 1
  spline S483 degree 3 poles (1.8965, 31.2232) (2.7191, 31.2232) (3.5417, 31.2232) (4.3893, 31.2232) knots 0 0 0 0 1 1 1 1
  spline S484 degree 3 poles (4.3893, 31.2232) (4.4857, 31.5413) (4.5821, 31.8594) (4.6814, 32.1872) knots 0 0 0 0 1 1 1 1
  spline S485 degree 3 poles (4.6814, 32.1872) (4.8112, 32.5991) (4.941, 33.0111) (5.0748, 33.4355) knots 0 0 0 0 1 1 1 1
  spline S486 degree 3 poles (5.0748, 33.4355) (5.202, 33.8462) (5.3293, 34.2568) (5.4604, 34.6799) knots 0 0 0 0 1 1 1 1
  spline S487 degree 3 poles (5.4604, 34.6799) (5.8849, 35.7102) (5.8849, 35.7102) (6.882, 36.2087) knots 0 0 0 0 1 1 1 1
  spline S488 degree 3 poles (6.882, 36.2087) (7.2272, 37.6096) (7.2272, 37.6096) (7.4429, 39.2312) knots 0 0 0 0 1 1 1 1
  spline S489 degree 3 poles (7.4429, 39.2312) (7.5265, 39.782) (7.61, 40.3328) (7.6961, 40.9002) knots 0 0 0 0 1 1 1 1
  spline S490 degree 3 poles (7.6961, 40.9002) (7.7565, 41.3263) (7.8169, 41.7524) (7.8792, 42.1914) knots 0 0 0 0 1 1 1 1
  spline S491 degree 3 poles (0.4008, -1.6815) (0.7299, -1.6815) (1.0589, -1.6815) (1.3979, -1.6815) knots 0 0 0 0 1 1 1 1
  spline S492 degree 3 poles (1.3979, -1.6815) (1.0635, -3.9694) (0.5199, -6.1314) (-0.1289, -8.3497) knots 0 0 0 0 1 1 1 1
  spline S493 degree 3 poles (-0.1289, -8.3497) (-0.3095, -8.9705) (-0.4901, -9.5914) (-0.6761, -10.231) knots 0 0 0 0 1 1 1 1
  spline S494 degree 3 poles (-0.6761, -10.231) (-0.8143, -10.7001) (-0.9525, -11.1693) (-1.0949, -11.6527) knots 0 0 0 0 1 1 1 1
  spline S495 degree 3 poles (-1.0949, -11.6527) (-0.7658, -11.6527) (-0.4368, -11.6527) (-0.0977, -11.6527) knots 0 0 0 0 1 1 1 1
  spline S496 degree 3 poles (-0.0977, -11.6527) (-0.2623, -12.3107) (-0.4268, -12.9688) (-0.5963, -13.6469) knots 0 0 0 0 1 1 1 1
  spline S497 degree 3 poles (-0.5963, -13.6469) (-1.9881, -13.6603) (-3.3798, -13.6702) (-4.7717, -13.678) knots 0 0 0 0 1 1 1 1
  spline S498 degree 3 poles (-4.7717, -13.678) (-5.1676, -13.6822) (-5.5635, -13.6864) (-5.9714, -13.6907) knots 0 0 0 0 1 1 1 1
  spline S499 degree 3 poles (-5.9714, -13.6907) (-8.9588, -13.7034) (-8.9588, -13.7034) (-10.0689, -13.1483) knots 0 0 0 0 1 1 1 1
  spline S500 degree 3 poles (-10.0689, -13.1483) (-10.9001, -13.3977) (-11.7313, -13.6475) (-12.5616, -13.9) knots 0 0 0 0 1 1 1 1
  spline S501 degree 3 poles (-12.5616, -13.9) (-14.7875, -14.4478) (-16.8229, -14.4674) (-18.9494, -13.5222) knots 0 0 0 0 1 1 1 1
  spline S502 degree 3 poles (-18.9494, -13.5222) (-20.8709, -11.985) (-20.8709, -11.985) (-21.5356, -10.6555) knots 0 0 0 0 1 1 1 1
  spline S503 degree 3 poles (-21.5356, -10.6555) (-21.4253, -8.5585) (-21.2114, -7.4271) (-20.04, -5.67) knots 0 0 0 0 1 1 1 1
  spline S504 degree 3 poles (-20.04, -5.67) (-20.0573, -6.0183) (-20.0747, -6.3666) (-20.0926, -6.7255) knots 0 0 0 0 1 1 1 1
  spline S505 degree 3 poles (-20.0926, -6.7255) (-20.1061, -7.1792) (-20.1196, -7.633) (-20.1335, -8.1004) knots 0 0 0 0 1 1 1 1
  spline S506 degree 3 poles (-20.1335, -8.1004) (-20.1508, -8.5516) (-20.1682, -9.0028) (-20.186, -9.4676) knots 0 0 0 0 1 1 1 1
  spline S507 degree 3 poles (-20.186, -9.4676) (-20.1378, -9.8596) (-20.0896, -10.2516) (-20.04, -10.6555) knots 0 0 0 0 1 1 1 1
  spline S508 degree 3 poles (-20.04, -10.6555) (-19.5464, -10.9846) (-19.0528, -11.3136) (-18.5443, -11.6527) knots 0 0 0 0 1 1 1 1
  spline S509 degree 3 poles (-18.5443, -11.6527) (-18.5443, -12.1462) (-18.5443, -12.6398) (-18.5443, -13.1483) knots 0 0 0 0 1 1 1 1
  spline S510 degree 3 poles (-18.5443, -13.1483) (-16.0765, -12.9838) (-13.6086, -12.8193) (-11.066, -12.6498) knots 0 0 0 0 1 1 1 1
  spline S511 degree 3 poles (-11.066, -12.6498) (-11.066, -12.3207) (-11.066, -11.9917) (-11.066, -11.6527) knots 0 0 0 0 1 1 1 1
  spline S512 degree 3 poles (-11.066, -11.6527) (-10.735, -11.8108) (-10.404, -11.9688) (-10.063, -12.1317) knots 0 0 0 0 1 1 1 1
  spline S513 degree 3 poles (-10.063, -12.1317) (-8.2695, -12.7554) (-6.557, -12.8751) (-4.6782, -12.9614) knots 0 0 0 0 1 1 1 1
  spline S514 degree 3 poles (-4.6782, -12.9614) (-4.1601, -12.9903) (-4.1601, -12.9903) (-3.6315, -13.0198) knots 0 0 0 0 1 1 1 1
  spline S515 degree 3 poles (-3.6315, -13.0198) (-2.7861, -13.0664) (-1.9405, -13.1079) (-1.0949, -13.1483) knots 0 0 0 0 1 1 1 1
  spline S516 degree 3 poles (-1.0949, -13.1483) (-1.4239, -12.9838) (-1.7529, -12.8193) (-2.092, -12.6498) knots 0 0 0 0 1 1 1 1
  spline S517 degree 3 poles (-2.092, -12.6498) (-1.9274, -10.84) (-1.7629, -9.0302) (-1.5934, -7.1656) knots 0 0 0 0 1 1 1 1
  spline S518 degree 3 poles (-1.5934, -7.1656) (-1.2644, -7.1656) (-0.9353, -7.1656) (-0.5963, -7.1656) knots 0 0 0 0 1 1 1 1
  spline S519 degree 3 poles (-0.5963, -7.1656) (-0.5963, -6.1785) (-0.5963, -5.1914) (-0.5963, -4.1743) knots 0 0 0 0 1 1 1 1
  spline S520 degree 3 poles (-0.5963, -4.1743) (-0.2673, -4.1743) (0.0618, -4.1743) (0.4008, -4.1743) knots 0 0 0 0 1 1 1 1
  spline S521 degree 3 poles (0.4008, -4.1743) (0.4008, -3.3517) (0.4008, -2.5291) (0.4008, -1.6815) knots 0 0 0 0 1 1 1 1
  spline S522 degree 3 poles (14.3604, 11.7795) (14.5249, 11.2859) (14.6894, 10.7923) (14.8589, 10.2838) knots 0 0 0 0 1 1 1 1
  spline S523 degree 3 poles (14.8589, 10.2838) (15.8561, 9.6811) (15.8561, 9.6811) (16.8532, 9.2867) knots 0 0 0 0 1 1 1 1
  spline S524 degree 3 poles (16.8532, 9.2867) (16.6886, 8.9577) (16.5241, 8.6286) (16.3546, 8.2896) knots 0 0 0 0 1 1 1 1
  spline S525 degree 3 poles (16.3546, 8.2896) (16.0256, 8.2896) (15.6965, 8.2896) (15.3575, 8.2896) knots 0 0 0 0 1 1 1 1
  spline S526 degree 3 poles (15.3575, 8.2896) (15.3575, 7.467) (15.3575, 6.6444) (15.3575, 5.7968) knots 0 0 0 0 1 1 1 1
  spline S527 degree 3 poles (15.3575, 5.7968) (14.8639, 5.55) (14.8639, 5.55) (14.3604, 5.2983) knots 0 0 0 0 1 1 1 1
  spline S528 degree 3 poles (14.3604, 5.2983) (13.8668, 4.5579) (13.8668, 4.5579) (13.3633, 3.8026) knots 0 0 0 0 1 1 1 1
  spline S529 degree 3 poles (13.3633, 3.8026) (13.1987, 4.2962) (13.0342, 4.7897) (12.8647, 5.2983) knots 0 0 0 0 1 1 1 1
  spline S530 degree 3 poles (12.8647, 5.2983) (12.5357, 5.4628) (12.2066, 5.6273) (11.8676, 5.7968) knots 0 0 0 0 1 1 1 1
  spline S531 degree 3 poles (11.8676, 5.7968) (11.8676, 6.9601) (11.8676, 8.1234) (11.8676, 9.2867) knots 0 0 0 0 1 1 1 1
  spline S532 degree 3 poles (11.8676, 9.2867) (11.5386, 9.4512) (11.2095, 9.6157) (10.8705, 9.7853) knots 0 0 0 0 1 1 1 1
  spline S533 degree 3 poles (10.8705, 9.7853) (10.706, 8.6336) (10.5414, 7.4819) (10.3719, 6.2954) knots 0 0 0 0 1 1 1 1
  spline S534 degree 3 poles (10.3719, 6.2954) (10.0429, 6.4599) (9.7138, 6.6244) (9.3748, 6.7939) knots 0 0 0 0 1 1 1 1
  spline S535 degree 3 poles (9.3748, 6.7939) (9.3748, 8.2746) (9.3748, 9.7553) (9.3748, 11.2809) knots 0 0 0 0 1 1 1 1
  spline S536 degree 3 poles (9.3748, 11.2809) (10.9774, 12.0822) (12.5836, 11.8081) (14.3604, 11.7795) knots 0 0 0 0 1 1 1 1
  spline S537 degree 3 poles (1.8965, 47.6755) (2.2255, 47.511) (2.5546, 47.3465) (2.8936, 47.177) knots 0 0 0 0 1 1 1 1
  spline S538 degree 3 poles (2.8936, 47.177) (2.7291, 46.6834) (2.5645, 46.1898) (2.395, 45.6813) knots 0 0 0 0 1 1 1 1
  spline S539 degree 3 poles (2.395, 45.6813) (2.8886, 45.3522) (3.3822, 45.0232) (3.8907, 44.6842) knots 0 0 0 0 1 1 1 1
  spline S540 degree 3 poles (3.8907, 44.6842) (3.7827, 44.2629) (3.7827, 44.2629) (3.6726, 43.8331) knots 0 0 0 0 1 1 1 1
  spline S541 degree 3 poles (3.6726, 43.8331) (3.2926, 42.2842) (2.9713, 40.7239) (2.6443, 39.1631) knots 0 0 0 0 1 1 1 1
  spline S542 degree 3 poles (2.6443, 39.1631) (2.395, 38.2029) (2.395, 38.2029) (1.8965, 37.7044) knots 0 0 0 0 1 1 1 1
  spline S543 degree 3 poles (1.8965, 37.7044) (1.139, 37.6686) (0.38, 37.6626) (-0.3782, 37.6732) knots 0 0 0 0 1 1 1 1
  spline S544 degree 3 poles (-0.3782, 37.6732) (-0.7901, 37.6777) (-1.2021, 37.6822) (-1.6265, 37.6869) knots 0 0 0 0 1 1 1 1
  spline S545 degree 3 poles (-1.6265, 37.6869) (-2.1037, 37.6955) (-2.1037, 37.6955) (-2.5905, 37.7044) knots 0 0 0 0 1 1 1 1
  spline S546 degree 3 poles (-2.5905, 37.7044) (-3.0891, 39.2001) (-3.0891, 39.2001) (-2.5905, 40.6957) knots 0 0 0 0 1 1 1 1
  spline S547 degree 3 poles (-2.5905, 40.6957) (-2.2615, 40.6957) (-1.9324, 40.6957) (-1.5934, 40.6957) knots 0 0 0 0 1 1 1 1
  spline S548 degree 3 poles (-1.5934, 40.6957) (-1.5934, 41.3538) (-1.5934, 42.0119) (-1.5934, 42.69) knots 0 0 0 0 1 1 1 1
  spline S549 degree 3 poles (-1.5934, 42.69) (-2.2515, 42.5254) (-2.9096, 42.3609) (-3.5876, 42.1914) knots 0 0 0 0 1 1 1 1
  spline S550 degree 3 poles (-3.5876, 42.1914) (-2.3673, 44.7846) (-0.3958, 46.091) (1.8965, 47.6755) knots 0 0 0 0 1 1 1 1
  spline S551 degree 3 poles (1.8965, 44.1856) (1.2149, 43.4849) (0.5534, 42.7646) (-0.0977, 42.0356) knots 0 0 0 0 1 1 1 1
  spline S552 degree 3 poles (-0.0977, 42.0356) (-0.4576, 41.6365) (-0.8175, 41.2374) (-1.1883, 40.8262) knots 0 0 0 0 1 1 1 1
  spline S553 degree 3 poles (-1.1883, 40.8262) (-2.1801, 39.722) (-2.1801, 39.722) (-2.5905, 38.2029) knots 0 0 0 0 1 1 1 1
  spline S554 degree 3 poles (-2.5905, 38.2029) (-0.595, 38.1572) (-0.595, 38.1572) (1.3979, 38.2029) knots 0 0 0 0 1 1 1 1
  spline S555 degree 3 poles (1.3979, 38.2029) (2.2652, 39.0702) (2.0819, 40.2937) (2.1769, 41.4747) knots 0 0 0 0 1 1 1 1
  spline S556 degree 3 poles (2.1769, 41.4747) (2.2187, 41.9792) (2.2605, 42.4837) (2.3035, 43.0035) knots 0 0 0 0 1 1 1 1
  spline S557 degree 3 poles (2.3035, 43.0035) (2.3337, 43.3936) (2.3639, 43.7837) (2.395, 44.1856) knots 0 0 0 0 1 1 1 1
  spline S558 degree 3 poles (2.395, 44.1856) (2.2305, 44.1856) (2.066, 44.1856) (1.8965, 44.1856) knots 0 0 0 0 1 1 1 1
  spline S559 degree 3 poles (-10.0689, 13.7737) (-10.0689, 13.4447) (-10.0689, 13.1156) (-10.0689, 12.7766) knots 0 0 0 0 1 1 1 1
  spline S560 degree 3 poles (-10.0689, 12.7766) (-11.8786, 12.6121) (-13.6884, 12.4475) (-15.553, 12.278) knots 0 0 0 0 1 1 1 1
  spline S561 degree 3 poles (-15.553, 12.278) (-15.2239, 11.4554) (-14.8949, 10.6328) (-14.5559, 9.7853) knots 0 0 0 0 1 1 1 1
  spline S562 degree 3 poles (-14.5559, 9.7853) (-14.4571, 6.3347) (-15.0153, 3.3823) (-16.5501, 0.3127) knots 0 0 0 0 1 1 1 1
  spline S563 degree 3 poles (-16.5501, 0.3127) (-16.6735, -0.1963) (-16.6735, -0.1963) (-16.7994, -0.7156) knots 0 0 0 0 1 1 1 1
  spline S564 degree 3 poles (-16.7994, -0.7156) (-17.1673, -2.1414) (-17.8648, -3.3729) (-18.5443, -4.6729) knots 0 0 0 0 1 1 1 1
  spline S565 degree 3 poles (-18.5443, -4.6729) (-18.8734, -4.6729) (-19.2024, -4.6729) (-19.5414, -4.6729) knots 0 0 0 0 1 1 1 1
  spline S566 degree 3 poles (-19.5414, -4.6729) (-19.7059, -5.0019) (-19.8705, -5.331) (-20.04, -5.67) knots 0 0 0 0 1 1 1 1
  spline S567 degree 3 poles (-20.04, -5.67) (-19.8124, -3.7358) (-19.3369, -1.9805) (-18.7118, -0.145) knots 0 0 0 0 1 1 1 1
  spline S568 degree 3 poles (-18.7118, -0.145) (-18.4747, 0.5525) (-18.4747, 0.5525) (-18.2327, 1.264) knots 0 0 0 0 1 1 1 1
  spline S569 degree 3 poles (-18.2327, 1.264) (-17.9017, 2.2253) (-17.5655, 3.1848) (-17.2239, 4.1424) knots 0 0 0 0 1 1 1 1
  spline S570 degree 3 poles (-17.2239, 4.1424) (-16.167, 7.2893) (-15.9381, 9.5047) (-16.5501, 12.7766) knots 0 0 0 0 1 1 1 1
  spline S571 degree 3 poles (-16.5501, 12.7766) (-15.7507, 12.9446) (-14.9508, 13.1103) (-14.1508, 13.2751) knots 0 0 0 0 1 1 1 1
  spline S572 degree 3 poles (-14.1508, 13.2751) (-13.7054, 13.3677) (-13.26, 13.4602) (-12.8012, 13.5556) knots 0 0 0 0 1 1 1 1
  spline S573 degree 3 poles (-12.8012, 13.5556) (-11.5645, 13.7737) (-11.5645, 13.7737) (-10.0689, 13.7737) knots 0 0 0 0 1 1 1 1
  spline S574 degree 3 poles (-33.501, 35.7102) (-33.1925, 35.3091) (-32.884, 34.9081) (-32.5662, 34.4949) knots 0 0 0 0 1 1 1 1
  spline S575 degree 3 poles (-32.5662, 34.4949) (-31.3585, 33.0386) (-31.0159, 32.7777) (-29.1698, 32.563) knots 0 0 0 0 1 1 1 1
  spline S576 degree 3 poles (-29.1698, 32.563) (-27.5506, 32.7158) (-27.0543, 32.9163) (-25.7422, 33.7471) knots 0 0 0 0 1 1 1 1
  spline S577 degree 3 poles (-25.7422, 33.7471) (-24.0284, 34.7131) (-24.0284, 34.7131) (-22.5639, 34.5884) knots 0 0 0 0 1 1 1 1
  spline S578 degree 3 poles (-22.5639, 34.5884) (-22.0549, 34.4033) (-22.0549, 34.4033) (-21.5356, 34.2145) knots 0 0 0 0 1 1 1 1
  spline S579 degree 3 poles (-21.5356, 34.2145) (-21.5668, 33.0927) (-21.5668, 33.0927) (-22.0342, 31.7217) knots 0 0 0 0 1 1 1 1
  spline S580 degree 3 poles (-22.0342, 31.7217) (-24.7908, 29.8299) (-27.5983, 28.5298) (-31.0082, 28.7304) knots 0 0 0 0 1 1 1 1
  spline S581 degree 3 poles (-31.0082, 28.7304) (-29.4686, 29.6101) (-28.8978, 29.7275) (-27.0198, 29.7275) knots 0 0 0 0 1 1 1 1
  spline S582 degree 3 poles (-27.0198, 29.7275) (-27.1843, 30.3856) (-27.3488, 31.0437) (-27.5183, 31.7217) knots 0 0 0 0 1 1 1 1
  spline S583 degree 3 poles (-27.5183, 31.7217) (-29.1636, 31.5572) (-30.8088, 31.3927) (-32.5039, 31.2232) knots 0 0 0 0 1 1 1 1
  spline S584 degree 3 poles (-32.5039, 31.2232) (-32.5039, 31.8813) (-32.5039, 32.5394) (-32.5039, 33.2174) knots 0 0 0 0 1 1 1 1
  spline S585 degree 3 poles (-32.5039, 33.2174) (-32.9975, 33.3819) (-33.491, 33.5464) (-33.9995, 33.7159) knots 0 0 0 0 1 1 1 1
  spline S586 degree 3 poles (-33.9995, 33.7159) (-33.835, 34.374) (-33.6705, 35.0321) (-33.501, 35.7102) knots 0 0 0 0 1 1 1 1
  spline S587 degree 3 poles (25.3286, -2.6786) (25.8222, -2.8432) (26.3158, -3.0077) (26.8243, -3.1772) knots 0 0 0 0 1 1 1 1
  spline S588 degree 3 poles (26.8243, -3.1772) (26.8243, -3.8353) (26.8243, -4.4934) (26.8243, -5.1714) knots 0 0 0 0 1 1 1 1
  spline S589 degree 3 poles (26.8243, -5.1714) (26.4952, -5.1714) (26.1662, -5.1714) (25.8272, -5.1714) knots 0 0 0 0 1 1 1 1
  spline S590 degree 3 poles (25.8272, -5.1714) (25.8272, -5.994) (25.8272, -6.8167) (25.8272, -7.6642) knots 0 0 0 0 1 1 1 1
  spline S591 degree 3 poles (25.8272, -7.6642) (25.3336, -7.6642) (24.84, -7.6642) (24.3315, -7.6642) knots 0 0 0 0 1 1 1 1
  spline S592 degree 3 poles (24.3315, -7.6642) (24.496, -8.8159) (24.6605, -9.9675) (24.8301, -11.1541) knots 0 0 0 0 1 1 1 1
  spline S593 degree 3 poles (24.8301, -11.1541) (26.064, -11.6477) (26.064, -11.6477) (27.3228, -12.1512) knots 0 0 0 0 1 1 1 1
  spline S594 degree 3 poles (27.3228, -12.1512) (27.3228, -12.3157) (27.3228, -12.4803) (27.3228, -12.6498) knots 0 0 0 0 1 1 1 1
  spline S595 degree 3 poles (27.3228, -12.6498) (28.639, -12.6498) (29.9552, -12.6498) (31.3113, -12.6498) knots 0 0 0 0 1 1 1 1
  spline S596 degree 3 poles (31.3113, -12.6498) (31.3113, -12.4852) (31.3113, -12.3207) (31.3113, -12.1512) knots 0 0 0 0 1 1 1 1
  spline S597 degree 3 poles (31.3113, -12.1512) (35.0148, -11.5102) (35.0148, -11.5102) (36.7954, -12.1512) knots 0 0 0 0 1 1 1 1
  spline S598 degree 3 poles (36.7954, -12.1512) (36.7954, -12.4803) (36.7954, -12.8093) (36.7954, -13.1483) knots 0 0 0 0 1 1 1 1
  spline S599 degree 3 poles (36.7954, -13.1483) (39.2633, -13.1483) (41.7311, -13.1483) (44.2737, -13.1483) knots 0 0 0 0 1 1 1 1
  spline S600 degree 3 poles (44.2737, -13.1483) (44.027, -12.1612) (44.027, -12.1612) (43.7752, -11.1541) knots 0 0 0 0 1 1 1 1
  spline S601 degree 3 poles (43.7752, -11.1541) (44.1042, -11.3186) (44.4333, -11.4831) (44.7723, -11.6527) knots 0 0 0 0 1 1 1 1
  spline S602 degree 3 poles (44.7723, -11.6527) (44.7723, -12.3107) (44.7723, -12.9688) (44.7723, -13.6469) knots 0 0 0 0 1 1 1 1
  spline S603 degree 3 poles (44.7723, -13.6469) (43.2974, -13.6603) (41.8226, -13.6702) (40.3476, -13.678) knots 0 0 0 0 1 1 1 1
  spline S604 degree 3 poles (40.3476, -13.678) (39.9279, -13.6822) (39.5083, -13.6864) (39.0759, -13.6907) knots 0 0 0 0 1 1 1 1
  spline S605 degree 3 poles (39.0759, -13.6907) (38.6742, -13.6923) (38.2726, -13.6939) (37.8587, -13.6956) knots 0 0 0 0 1 1 1 1
  spline S606 degree 3 poles (37.8587, -13.6956) (37.3026, -13.6995) (37.3026, -13.6995) (36.7353, -13.7035) knots 0 0 0 0 1 1 1 1
  spline S607 degree 3 poles (36.7353, -13.7035) (35.7983, -13.6469) (35.7983, -13.6469) (34.8012, -13.1483) knots 0 0 0 0 1 1 1 1
  spline S608 degree 3 poles (34.8012, -13.1483) (34.2768, -13.3026) (33.7523, -13.4568) (33.212, -13.6157) knots 0 0 0 0 1 1 1 1
  spline S609 degree 3 poles (33.212, -13.6157) (30.5857, -14.3476) (28.7126, -14.5154) (26.1699, -13.4599) knots 0 0 0 0 1 1 1 1
  spline S610 degree 3 poles (26.1699, -13.4599) (24.8301, -12.6498) (24.8301, -12.6498) (23.8329, -11.6527) knots 0 0 0 0 1 1 1 1
  spline S611 degree 3 poles (23.8329, -11.6527) (23.3135, -8.462) (24.1598, -5.6216) (25.3286, -2.6786) knots 0 0 0 0 1 1 1 1
  spline S612 degree 3 poles (5.8849, -6.6671) (6.8197, -6.7606) (6.8197, -6.7606) (7.8792, -7.1656) knots 0 0 0 0 1 1 1 1
  spline S613 degree 3 poles (7.8792, -7.1656) (9.0421, -9.1039) (8.8785, -10.4963) (8.3777, -12.6498) knots 0 0 0 0 1 1 1 1
  spline S614 degree 3 poles (8.3777, -12.6498) (8.8713, -12.8143) (9.3649, -12.9788) (9.8734, -13.1483) knots 0 0 0 0 1 1 1 1
  spline S615 degree 3 poles (9.8734, -13.1483) (4.1292, -13.8127) (4.1292, -13.8127) (1.3979, -13.1483) knots 0 0 0 0 1 1 1 1
  spline S616 degree 3 poles (1.3979, -13.1483) (1.7784, -12.7884) (2.1588, -12.4285) (2.5508, -12.0577) knots 0 0 0 0 1 1 1 1
  spline S617 degree 3 poles (2.5508, -12.0577) (4.1642, -10.3694) (5.1483, -8.877) (5.8849, -6.6671) knots 0 0 0 0 1 1 1 1
  spline S618 degree 3 poles (-17.0486, 46.1798) (-16.8841, 46.1798) (-16.7196, 46.1798) (-16.5501, 46.1798) knots 0 0 0 0 1 1 1 1
  spline S619 degree 3 poles (-16.5501, 46.1798) (-16.4526, 45.1416) (-16.36, 44.1028) (-16.2697, 43.0639) knots 0 0 0 0 1 1 1 1